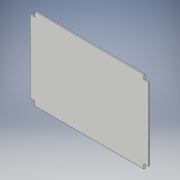
# Autodesk Inventor part: arm_enclosure_top_panel
Saved by Autodesk Inventor 2019 (Build 230136000, 136)
## iProperties
Created: 2018-07-20
Part Number: arm_enclosure_top_panel
Material: Generic
Document SubType Name: Modeling
Designer: Brian
Density: 1 g/cm^3
Appearance: Default
Author: Brian
Autodesk Inventor part; units mm, degrees
ref_plane "YZ Plane" through (0, 0, 0) normal (1, 0, 0) x (0, 1, 0)
ref_plane "XZ Plane" through (0, 0, 0) normal (0, 1, 0) x (-1, 0, 0)
ref_plane "XY Plane" through (0, 0, 0) normal (0, 0, 1) x (1, 0, 0)
sketch "Sketch1" plane through (0, 0, 0) normal (0, 0, 1) x (1, 0, 0)
  line L0 (0, 0) -> (25.4, 0)
  line L1 (25.4, 406.4) -> (0, 406.4)
  line L2 (0, 406.4) -> (0, 0)
  line L3 (635, 406.4) -> (635, 431.8)
  line L4 (635, 431.8) -> (25.4, 431.8)
  line L5 (25.4, 431.8) -> (25.4, 406.4)
  line L6 (635, 406.4) -> (660.4, 406.4)
  line L7 (660.4, 406.4) -> (660.4, 0)
  line L8 (660.4, 0) -> (635, 0)
  line L9 (25.4, 0) -> (25.4, -25.4)
  line L10 (25.4, -25.4) -> (635, -25.4)
  line L11 (635, -25.4) -> (635, 0)
  dimension "d0" = 406.4
  dimension "d1" = 25.4
  dimension "d2" = 609.6
  constraints: 24 end point, 7 equal length, 6 parallel, 3 perpendicular, 3 point on line, 2 horizontal
  measures "d0" distance of L1.end L0.start
  measures "d1" distance of L3.start L3.end
  measures "d2" distance of L3.end L4.end
extrude "Extrusion1" add sketch "Sketch1" along normal blind 6.35
body "Solid1"
